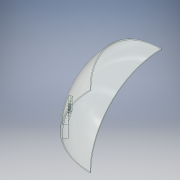
# Autodesk Inventor part: shell
Saved by Autodesk Inventor 2019 (Build 230136000, 136)
## iProperties
Created: 2019-02-10
Part Number: shell
Material: Glass
Document SubType Name: Modeling
Designer: mashimaro
Density: 2.18 g/cm^3
Appearance: Clear
Author: mashimaro
Autodesk Inventor part; units mm, degrees
ref_plane "YZ Plane" through (0, 0, 0) normal (1, 0, 0) x (0, 1, 0)
ref_plane "XZ Plane" through (0, 0, 0) normal (0, 1, 0) x (-1, 0, 0)
ref_plane "XY Plane" through (0, 0, 0) normal (0, 0, 1) x (1, 0, 0)
sketch "Sketch1" plane through (0, 0, 0) normal (0, 1, 0) x (-1, 0, 0)
  arc A0 (172, 0) -> (0, 172) centre (0, 0) ccw
  line L0 (0, 172) -> (0, 0)
  line L1 (172, 0) -> (0, 0)
  constraints: 4 end point, 2 point on circle, 1 centre point, 1 horizontal, 1 vertical
revolve "Revolution1" add sketch "Sketch1" angle 90 about axis through (0, 0, 172) along (0, 0, -1)
sketch "Sketch2" plane through (-172, 0, 0) normal (0, -1, 0) x (1, 0, 0)
  arc A0 (172, 170) -> (2, 0) centre (172, 0) ccw
  line L0 (172, 0) -> (172, 172) projected
  line L1 (172, 0) -> (2, 0)
  line L2 (172, 0) -> (172, 170)
  constraints: 4 end point, 2 point on circle, 1 centre point, 1 coincident, 1 perpendicular, 1 point on line
revolve "Revolution2" cut sketch "Sketch2" angle 90 about axis through (0, 0, 0) along (0, 0, -1)
sketch "Sketch4" plane through (0, 0, 0) normal (0, -1, 0) x (0.7071068, 0, -0.7071068)
  arc A0 (-120.2082, 120.2082) -> (-120.2082, -120.2082) centre (0, 0) ccw projected
  line L0 (-170, 0) -> (-150, 0)
  line L1 (-150, 0) -> (-150, -20)
  line L2 (-150, 0) -> (-150, 20)
  line L3 (-150, -20) -> (-170, -20)
  line L4 (-170, -20) -> (-170, 20)
  line L5 (-170, 20) -> (-150, 20)
  dimension "d34" = 20
  dimension "d35" = 20
  dimension "d36" = 20
  dimension "d56" = 20
  dimension "d57" = 40
  constraints: 12 end point, 2 horizontal, 2 perpendicular, 1 point on circle, 1 vertical
  measures "d34" distance of L0.start L0.end
  measures "d35" distance of L0.end L1.end
  measures "d36" distance of L0.end L2.end
  measures "d56" distance of L1.end L3.end
  measures "d57" distance of L3.end L4.end
extrude "Extrusion2" add sketch "Sketch4" against normal blind 60
sketch "Sketch6" plane through (0, 0, 0) normal (1, 0, 0) x (0, -0.7071068, -0.7071068)
  line L0 (-120.2082, 120.2082) -> (0, 0) projected
  line L1 (-120.2082, -120.2082) -> (-121.6224, -121.6224) projected
  arc A0 (-121.6224, 121.6224) -> (-121.6224, -121.6224) centre (0, 0) ccw
  line L2 (0, 0) -> (-120.2082, -120.2082) projected
  arc A1 (-134.3503, 134.3503) -> (-134.3503, -134.3503) centre (0, 0) ccw
  line L3 (-121.6224, 121.6224) -> (-134.3503, 134.3503)
  line L4 (-121.6224, -121.6224) -> (-134.3503, -134.3503)
  point P0 (-74.4097, -74.4097)
  constraints: 4 end point, 4 point on circle, 2 centre point, 2 coincident, 1 perpendicular
revolve "Revolution3" cut sketch "Sketch6" angle 90 about axis through (0, 170, 0) along (0, -1, 0)
sketch "Sketch9" plane through (-120.2082, 0, 91.9239) normal (-0.7071068, 0, -0.7071068) x (-0.7071068, 0, 0.7071068)
  line L0 (0, 0) -> (0, 60) projected
  line L1 (0, 0) -> (8, 0)
  line L2 (18.8194, 0) -> (0, 0) projected
  line L3 (8, 0) -> (8, 35)
  line L4 (8, 35) -> (1.5295, 59.1481)
  line L5 (1.5295, 59.1481) -> (4.7087, 60)
  line L6 (0, 60) -> (7.7973, 60) projected
  line L7 (4.7087, 60) -> (0, 60)
  line L8 (0, 60) -> (0, 0)
  point P0 (-150, 0)
  dimension "d58" = 8
  dimension "d59" = 35
  dimension "d60" = 25
  dimension "d61" = 165
  constraints: 12 end point, 2 perpendicular, 2 point on line, 1 horizontal
  measures "d58" distance of L0.start L1.end
  measures "d59" distance of L1.end L3.end
  measures "d60" distance of L3.end L4.end
  measures "d61" angle of L4 L3
extrude "Extrusion5" cut sketch "Sketch9" against normal blind 40
sketch "Sketch10" plane through (-125.865, 35, 97.5807) normal (0.6830127, -0.258819, -0.6830127) x (-0.7071068, 0, -0.7071068)
  line L0 (0, 25) -> (0, 0) projected
  line L1 (0, 25) -> (-40, 25) projected
  line L2 (-40, 0) -> (-40, 25) projected
  line L3 (-40, 25) -> (0, 25) projected
  circle A0 centre (-20, 12.5) radius 4
  circle A1 centre (-15.0503, 7.5503) radius 1
  circle A2 centre (-24.9497, 7.5503) radius 1
  circle A3 centre (-24.9497, 17.4497) radius 1
  circle A4 centre (-15.0503, 17.4497) radius 1
  line L4 (-24.9497, 7.5503) -> (-10.9497, 7.5503) construction
  circle A5 centre (-29.8995, 12.5) radius 4
  circle A6 centre (-34.8492, 7.5503) radius 1
  circle A7 centre (-34.8492, 17.4497) radius 1
  line L5 (-15.0503, 17.4497) -> (-1.0503, 17.4497) construction
  line L6 (-15.0503, 7.5503) -> (-1.0503, 7.5503) construction
  circle A8 centre (-10.1005, 12.5) radius 4
  circle A9 centre (-5.1508, 7.5503) radius 1
  circle A10 centre (-5.1508, 17.4497) radius 1
  dimension "d64" = 8
  dimension "d68" = 2
  dimension "d69" = 2
  dimension "d70" = 2
  dimension "d72" = 2
  dimension "d76" = 8
  dimension "d77" = 2
  dimension "d78" = 2
  dimension "d83" = 8
  dimension "d84" = 2
  dimension "d85" = 2
  constraints: 11 centre point, 6 end point, 3 horizontal
  measures "d64" diameter of A0
  measures "d68" diameter of A1
  measures "d69" diameter of A2
  measures "d70" diameter of A3
  measures "d72" diameter of A4
  measures "d76" diameter of A5
  measures "d77" diameter of A6
  measures "d78" diameter of A7
  measures "d83" diameter of A8
  measures "d84" diameter of A9
  measures "d85" diameter of A10
extrude "Extrusion6" cut sketch "Sketch10" against normal blind 3
body "Solid1"
